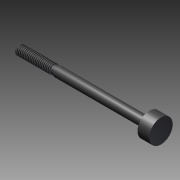
# Autodesk Inventor part: CJ2B10-15Z_ROD
Saved by Autodesk Inventor 2011 SP1 (Build 150282100, 282)
## iProperties
Created: 2018-06-19
Part Number: CJ2B10-15Z_ROD
Catalog Web Link: www.cadenas.de
Description: CJ2-Z ROD-Air Cylinder/Standard: Double Acting Single Rod
Vendor: SMC
Document SubType Name: Modeling
Designer: psAdmin
Manufacturer: SMC
Mass: 1.08304 g
Surface Area: 10.1292 cm^2
Volume: 1.08304 cm^3
Density: 1 g/cm^3
Category: PARTsolutions
Company: SMC
Title: CJ2B10-15Z_ROD
Author: Cadenas PARTsolutions
Comments: Air Cylinder/Standard: Double Acting Single Rod
PSOL_IDENT_0: {$CADENAS_DATA\23d-libs\smc_jp\actuator\standard_air_cylinder\cj2\cj2_z\parts\cj2_z_rod.prj},193 {VT
PSOL_IDENT_1: YP=3D},{NB=CJ2B10-15Z_ROD},{LINA=CJ2B10-15Z_ROD},{NN=CJ2-Z ROD},{DATE=15.05.2018 04:58:42},{GEOMDATE=
PSOL_IDENT_2: 24.06.2016 04:37:00},{VERSION=},{LINEID=370},{LINESUBID=-1},{WBVAR=STROKE,CUSHION,RODB}  {NB=CJ2B10-
PSOL_IDENT_3: 15Z_ROD},{LINA=CJ2B10-15Z_ROD},{KT=DUMMY},{ORDER=CJ2B10-15Z},{BORE=10},{MOUNT=(B) Basic},{MOUNTX=B},
PSOL_IDENT_4: {STROKE=15},{CUSHION=},{RODB=},{A=15},{D=4},{H=28},{MM=M4x0.7},{MM1=4},{MM2=0.7},{NA=12.5},{NA1=12.5
PSOL_IDENT_5: },{NA2=21.000},{S=46},{S1=46.000},{S2=65.000},{NB1=9.500},{SMAX=400.000},{P=8},{P1=8.000},{P2=8.000}
PSOL_IDENT_6: ,{P3=8.000}
NN: CJ2-Z ROD
NT: Air Cylinder/Standard: Double Acting Single Rod
NB: CJ2B10-15Z_ROD
NBSYN: $ORDER._ROD
LINA: CJ2B10-15Z_ROD
BORE: 10
MOUNT: (B) Basic
STROKE: 15
CUSHION: (-) Rubber cushion
RODB: (-) None
A: 15
D: 4
H: 28
MM: M4x0.7
MM1: 4
MM2: 0.7
NA1: 12.5
NA2: 21.000
S1: 46.000
S2: 65.000
NB1: 9.500
SMAX: 400.000
P1: 8.000
P2: 8.000
P3: 8.000
SUPPLIER: SMC
ARTICLENO: CJ2B10-15Z_ROD
BOMINFO: CJ2B10-15Z_ROD
CREATOR: CADENAS GmbH
Autodesk Inventor part; units mm, degrees
sketch "Sketch_2" plane through (0, 0, 0) normal (0, 0, 1) x (1, 0, 0)
  line L0 (60.5, 0) -> (0, 0)
  line L1 (0, 0) -> (0, 1.5705)
  line L2 (0, 1.5705) -> (0.4295, 2)
  line L3 (0.4295, 2) -> (15, 2)
  line L4 (15, 2) -> (15, 1.65)
  line L5 (15, 1.65) -> (16.5, 1.65)
  line L6 (16.5, 1.65) -> (16.5, 2)
  line L7 (16.5, 2) -> (55.5, 2)
  line L8 (55.5, 2) -> (55.5, 5)
  line L9 (55.5, 5) -> (60.5, 5)
  line L10 (60.5, 5) -> (60.5, 0)
  line L11 (60.5, 0) -> (0, 0)
  constraints: 24 end point
revolve "Revolution1" add sketch "Sketch_2" angle 360 about axis through (60.5, 0, 0) along (1, 0, 0)
thread "Thread1" size "M4x0.7" class "6g" standard "ISO Metric profile" full length
ref_plane "ROD_BA_XY" through (8, 0, 0) normal (-1, 0, 0) x (0, 0, -1)
ref_plane "ROD_BA_YZ" through (8, 0, 0) normal (0, 0, -1) x (0, -1, 0)
ref_plane "ROD_BA_ZX" through (8, 0, 0) normal (0, -1, 0) x (-1, 0, 0)
ref_plane "ROD_BODY_XY" through (28, 0, 0) normal (-1, 0, 0) x (0, 0, -1)
ref_plane "ROD_BODY_YZ" through (28, 0, 0) normal (0, 0, -1) x (0, -1, 0)
ref_plane "ROD_BODY_ZX" through (28, 0, 0) normal (0, -1, 0) x (-1, 0, 0)
ref_plane "rodnt1_XY" through (7.5, 0, 0) normal (1, 0, 0) x (0, 0, -1)
ref_plane "rodnt1_YZ" through (7.5, 0, 0) normal (0, 0, -1) x (0, 1, 0)
ref_plane "rodnt1_ZX" through (7.5, 0, 0) normal (0, 1, 0) x (1, 0, 0)
body "Solid1"
